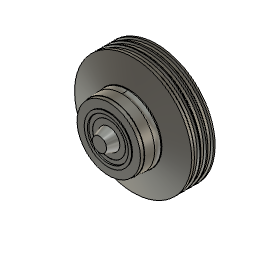
Suspension (Autodesk Fusion 360 design; units mm, degrees)
Autodesk Fusion 360 part; units mm, degrees
note: some values were not read from the file. Set by a fixed rule: which sketch regions a step uses.
sketch "Sketch1" plane through (0, 0, 0) normal (1, 0, 0) x (0, 1, 0) in component "Hind Drum "
  line L0 (0, 0) -> (0, 20.9296)
  line L1 (0, 20.9296) -> (-3.1394, 20.9296)
  line L2 (-10.988, 18.3134) -> (-5.7556, 18.3134)
  line L3 (-5.7556, 18.3134) -> (-3.1394, 20.9296)
  line L4 (-10.988, 18.3134) -> (-8.3718, 18.3134) construction
  line L5 (-8.3718, 18.3134) -> (-8.3718, 26.3527) construction
  line L6 (-10.988, 18.3134) -> (-13.6042, 20.9296)
  line L7 (-13.6042, 20.9296) -> (-16.2204, 20.9296)
  line L8 (-16.2204, 20.9296) -> (-18.8366, 18.3134)
  line L9 (-18.8366, 18.3134) -> (-24.069, 18.3134)
  line L10 (-24.069, 18.3134) -> (-26.6852, 20.9296)
  line L11 (-26.6852, 20.9296) -> (-28.255, 20.9296)
  line L12 (-28.255, 20.9296) -> (-31.0112, 18.3172)
  line L13 (-31.0112, 18.3172) -> (-36.2436, 18.3172)
  line L14 (-36.2436, 18.3172) -> (-38.7198, 20.9296)
  line L15 (-38.7198, 20.9296) -> (-43.9168, 20.9296)
  line L16 (0, 0) -> (-3.7685, 0)
  line L17 (-3.7685, 0) -> (-9.4336, 9.8123)
  line L18 (-9.4336, 9.8123) -> (-25.1308, 9.8123)
  line L19 (-34.5579, -88.9394) -> (-107.1355, -88.9394)
  line L20 (-107.1355, -88.9394) -> (-107.1355, -75.4982)
  line L21 (-107.1355, -75.4982) -> (-89.1773, -68.7615)
  line L22 (-89.1773, -68.7615) -> (-89.1807, -58.1112)
  line L23 (-89.1807, -58.1112) -> (-88.9739, -58.1112)
  line L24 (-88.9739, -58.1112) -> (-88.9762, -50.884)
  line L25 (-88.9762, -50.884) -> (-91.2673, -50.4985)
  line L26 (-91.2673, -50.4985) -> (-91.2692, -44.494)
  line L27 (-91.2692, -44.494) -> (-89.6864, -44.494)
  line L28 (-30.7894, 0.0114) -> (-25.1308, 9.8123)
  line L29 (-30.7894, 0.0114) -> (-34.5579, 0.0114)
  line L30 (-34.5579, 0.0114) -> (-34.5579, -88.9394)
  line L31 (-89.6864, -44.494) -> (-89.6864, -29.1366) construction
  line L32 (-89.6864, -44.494) -> (-89.6864, -29.1366)
  line L33 (-43.9168, 20.9296) -> (-52.5788, -26.3177)
  line L34 (-89.6864, -29.1366) -> (-90.3623, -29.1833)
  line L35 (-90.3623, -29.1833) -> (-90.1625, -29.512)
  line L36 (-90.1625, -29.512) -> (-83.1057, -29.0238)
  line L37 (-83.1057, -29.0238) -> (-82.7918, -28.474)
  line L38 (-82.7918, -28.474) -> (-65.5779, -27.2832)
  line L39 (-65.5779, -27.2832) -> (-65.1468, -27.2534)
  spline S0 degree 5 poles (-65.1468, -27.2534) (-65.066, -27.3424) (-64.8912, -27.5103) (-64.5889, -27.7318) (-64.1045, -27.9656) (-63.356, -28.1495) (-62.4566, -28.219) (-61.4038, -28.1724) (-60.2075, -28.017) (-58.8821, -27.7639) (-57.4422, -27.424) (-56.2081, -27.0898) (-55.2397, -26.8067) (-54.5753, -26.6038) (-54.2384, -26.4988) knots 0 0 0 0 0 0 0.1 0.2 0.3 0.4 0.5 0.6 0.7 0.8 0.9 1 1 1 1 1 1
  line L40 (-54.2384, -26.4988) -> (-52.5788, -26.3177)
  point P0 (-62.5199, -28.1882)
  dimension "d14" = 120
  dimension "d24" = 120
  constraint coincident L0.start L16.start
  constraint vertical L0
  constraint perpendicular L0 L1
  constraint horizontal L2
  constraint midpoint L2 L4.end
  constraint perpendicular L2 L5
  constraint horizontal L7
  constraint horizontal L9
  constraint equal L3 L8
  constraint horizontal L11
  constraint parallel L11 L13
  constraint horizontal L15
  constraint perpendicular L0 L16
  constraint horizontal L18
  constraint horizontal L19
  constraint perpendicular L19 L20
  constraint perpendicular L22 L23
  constraint perpendicular L23 L24
  constraint perpendicular L23 L26
  constraint horizontal L29
  constraint equal L16 L29
  constraint coincident L18.end L28.end
  constraint perpendicular L29 L30
  constraint coincident L29.end L30.start
  constraint perpendicular L27 L31
  measures "d14" angle of L16 L17
  measures "d24" angle of L28 L29
revolve "Revolve1" add sketch "Sketch1" angle 360 about axis through (0, -34.5579, -88.9394) along (0, -1, 0) contours L0 L1 L2 L3 L6 L7 L8 L9 L10 L11 L12 L13 L14 L15 L16 L17 L18 L19 L20 L21 L22 L23 L24 L25 L26 L27 L28 L29 L30 L32 L33 L36 L37 L38 L39 S0 L40 in component "Hind Drum "
move_body "Move1" bodies 1 to x (1, 0, 0) y (0, 1, 0) z (0, 0, 1) at (0, 107.1355, 88.9394) in component "Hind Drum "
component "Hind Drum " placed x (1, 0, 0) y (0, 1, 0) z (0, 0, 1) at (0, 0, 0)
component "Hind Drum " placed x (1, 0, 0) y (0, 1, 0) z (0, 0, 1) at (172.2981, 542.1576, 0)
